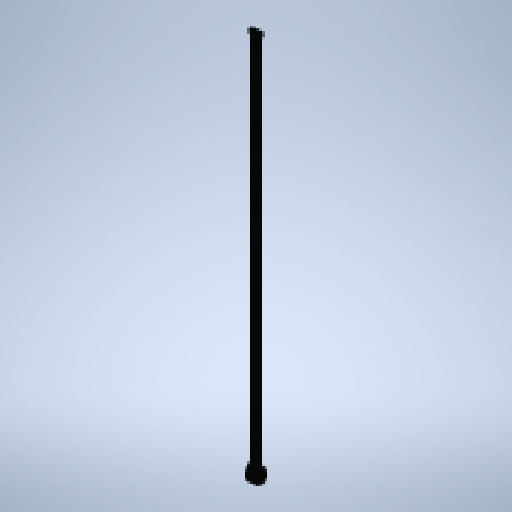
# Autodesk Inventor part: strap
Saved by Autodesk Inventor 2024 (Build 280153000, 153)
## iProperties
Created: 2023-05-23
Part Number: strap
Material: Nylon, molybdenum disulphide
Document SubType Name: Modeling
Designer: Patrick
Density: 1.13 g/cm^3
Appearance: Anodized - Black
Author: Patrick
Autodesk Inventor part; units mm, degrees
ref_plane "YZ Plane" through (0, 0, 0) normal (1, 0, 0) x (0, 1, 0)
ref_plane "XZ Plane" through (0, 0, 0) normal (0, 1, 0) x (-1, 0, 0)
ref_plane "XY Plane" through (0, 0, 0) normal (0, 0, 1) x (1, 0, 0)
sketch "Sketch1" plane through (0, 0, 0) normal (1, 0, 0) x (0, 1, 0)
  arc A0 (-16, 0) -> (16, 0) centre (0, 0) ccw
  arc A1 (-18, 0) -> (11.5702, -13.7888) centre (0, 0) ccw
  line L0 (11.5702, -13.7888) -> (25.6195, -2)
  line L1 (25.6195, -2) -> (800.1018, -2)
  arc A2 (801.81, 0) -> (811.81, 0) centre (806.81, 0) ccw
  arc A3 (800.1018, -2) -> (813.81, 0) centre (806.81, 0) ccw
  line L2 (-16, 0) -> (-18, 0)
  line L3 (813.81, 0) -> (811.81, 0)
  line L4 (801.81, 0) -> (16, 0)
  dimension "d0" = 32
  dimension "d1" = 5
  dimension "d2" = 2
  dimension "d3" = 2
  dimension "d4" = 2
  dimension "d5" = 40
  dimension "length" = 806.81
  constraints: 10 end point, 8 point on circle, 4 centre point, 4 horizontal, 3 coincident, 3 horizontal alignment, 1 tangent
  measures "d0" diameter of A0
  measures "d1" radius of A2
  measures "d2" radial gap between concentric circles of A3 A2
  measures "d3" radial gap between concentric circles of A0 A1
  measures "d4" distance between parallel lines of L4 L1
  measures "d5" angle of L4 L0
  measures "length" distance of point (0, 0) A2.centre
extrude "Extrusion1" add sketch "Sketch1" along normal mid plane 25.4
mirror "Mirror1" about plane through (0, 0, 0) normal (0, 0, 1) of "Extrusion1"
equation "\"d3\" = d2"
equation "\"d4\" = d2"
body "Solid1"
